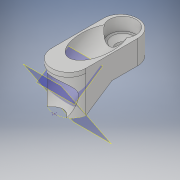
# Autodesk Inventor part: cable_cap
Saved by Autodesk Inventor 2019 (Build 230136000, 136)
## iProperties
Created: 2019-04-25
Part Number: cable_cap
Material: Generic
Document SubType Name: Modeling
Designer: assman
Density: 1 g/cm^3
Appearance: Default
Author: assman
## iProperties of the stored document cable_cap_3DPrint.ipt
Created: 2019-04-25
Part Number: cable_cap_3DPrint
Material: Generic
Document SubType Name: Modeling
Designer: assman
Density: 1 g/cm^3
Appearance: Default
Author: assman
Autodesk Inventor part; units mm, degrees
ref_plane "YZ Plane" through (0, 0, 0) normal (1, 0, 0) x (0, 1, 0)
ref_plane "XZ Plane" through (0, 0, 0) normal (0, 1, 0) x (-1, 0, 0)
ref_plane "XY Plane" through (0, 0, 0) normal (0, 0, 1) x (1, 0, 0)
sketch "Sketch1" plane through (0, 0, 0) normal (0, 1, 0) x (-1, 0, 0)
  line L0 (0, 10) -> (0, 10)
  line L1 (-4, 6) -> (-4, -6)
  line L2 (0, -10) -> (0, -10)
  line L3 (4, -6) -> (4, 6)
  line L4 (4, 10) -> (-4, -10) construction
  line L5 (-4, 10) -> (4, -10) construction
  circle A0 centre (0, -6.5) radius 1.5
  arc A1 (0, -10) -> (4, -6) centre (0, -6) ccw
  arc A2 (-4, -6) -> (0, -10) centre (0, -6) ccw
  arc A3 (4, 6) -> (0, 10) centre (0, 6) ccw
  arc A4 (0, 10) -> (-4, 6) centre (0, 6) ccw
  point P0 (0, 0)
  dimension "d0" = 8
  dimension "d1" = 20
  dimension "d2" = 3
  dimension "d3" = 3.5
  dimension "d4" = 4
  constraints: 12 end point, 8 point on circle, 8 point on line, 8 tangent, 5 centre point, 3 equal radius, 2 midpoint, 2 parallel, 1 horizontal, 1 perpendicular
  measures "d0" distance of L5.end L4.end
  measures "d1" distance of L4.end L5.start
  measures "d2" diameter of A0
  measures "d3" distance from line of L2 A0.centre
  measures "d4" radius of A1
extrude "Extrusion1" add sketch "Sketch1" along normal blind 5.5
sketch "Sketch2" plane through (0, 0, 0) normal (0, -1, 0) x (1, 0, 0)
  circle A0 centre (0, -6.5) radius 1.5 construction
  line L0 (-4, -6) -> (-4, 6) construction
  arc A1 (-4, -6) -> (4, -6) centre (0, -6) ccw construction
  line L1 (4, 6) -> (4, -6) construction
  arc A2 (4, 6) -> (-4, 6) centre (0, 6) ccw construction
  arc A3 (4, 6) -> (-4, 6) centre (0, 6) ccw projected
  arc A4 (4, 6) -> (-4, 6) centre (0, 5.2831) ccw
  point P0 (0, 0)
  constraints: 3 point on circle, 1 centre point
extrude "Extrusion2" cut sketch "Sketch2" against normal blind 4.5
sketch "Sketch4" plane through (0, 0, 0) normal (0, -1, 0) x (1, 0, 0)
  arc A0 (4, 6) -> (-4, 6) centre (0, 5.2831) ccw projected
  line L0 (-4, -6) -> (-4, 6) projected
  arc A1 (-4, -6) -> (4, -6) centre (0, -6) ccw projected
  line L1 (4, 6) -> (4, -6) projected
  circle A2 centre (0, -6.5) radius 1.5 projected
  point P0 (0, 0)
extrude "Extrusion3" add sketch "Sketch4" along normal blind 4
sketch "Sketch6" plane through (0, -4, 0) normal (0, -1, 0) x (1, 0, 0)
  circle A0 centre (0, -6.5) radius 1.5 projected
  arc A1 (-4, -6) -> (4, -6) centre (0, -6) ccw projected
  line L0 (4, 0) -> (4, -6)
  line L1 (4, 0) -> (-4, 0)
  arc A2 (-4, -6) -> (4, -6) centre (0, -6) ccw projected
  line L2 (-4, 0) -> (-4, -6)
  point P0 (0, 0)
  constraints: 6 end point, 1 tangent, 1 vertical
extrude "Extrusion4" cut sketch "Sketch6" against normal blind 4
sketch "Sketch7" plane through (-4, 5.5, -6) normal (-1, 0, 0) x (0, 0, 1)
  line L0 (12, -9.5) -> (15.3469, -9.5) projected
  line L1 (6, -9.5) -> (12, -9.5) projected
  line L2 (12, -9.5) -> (6, -9.5)
  line L3 (6, -5.5) -> (6, -9.5) projected
  line L4 (6, -9.5) -> (6, -5.5)
  line L5 (12, -9.5) -> (12, -1) projected
  line L6 (6, -5.5) -> (12, -9.5)
  constraints: 6 end point, 2 collinear
extrude "Extrusion5" cut sketch "Sketch7" against normal through all
ref_plane "Work Plane1" through (-4, 0.1603, 8.7735) normal (0, -0.8320503, -0.5547002) x (1, 0, 0)
sketch "Sketch8" plane through (0, -4, 0) normal (0, -1, 0) x (1, 0, 0)
  line L0 (-4, 6) -> (4, 6) construction
  arc A0 (4, 6) -> (-4, 6) centre (0, 5.2831) ccw construction
  point P0 (0, 0)
  point P1 (0, 9.3469)
  constraints: 1 point on circle
ref_plane "Work Plane3" through (-2, -4, 6) normal (0, 0.5547002, -0.8320503) x (1, 0, 0)
sketch "Sketch10" plane through (-2, -4, 6) normal (0, 0.5547002, -0.8320503) x (1, 0, 0)
  circle A0 centre (2, -4.3065) radius 3.55
  point P0 (2, 0)
  dimension "d18" = 7.1
  constraints: 1 centre point
  measures "d18" diameter of A0
extrude "Extrusion6" cut sketch "Sketch10" along normal blind 20 and the other way blind 10
sketch "Sketch11" plane through (0, 5.5, 0) normal (0, 1, 0) x (1, 0, 0)
  arc A0 (1.4864, 6.2983) -> (-1.4864, 6.2983) centre (0, 6.5) ccw construction
  circle A1 centre (0, 6.5) radius 3.1
  point P0 (0, 0)
  dimension "d23" = 6.2
  constraints: 1 centre point, 1 coincident
  measures "d23" diameter of A1
extrude "Extrusion7" cut sketch "Sketch11" against normal blind 3
chamfer "Chamfer1" distance 1 angle 45 1 edges at (1.5, 2.5, -6.5)
body "Solid1"
